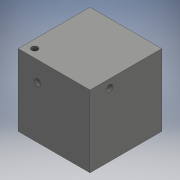
# Autodesk Inventor part: Bundhjørne1
Saved by Autodesk Inventor 2018 (Build 220112000, 112)
## iProperties
Created: 2018-01-29
Part Number: Bundhjørne1
Material: PC/ABS Plastic
Document SubType Name: Modeling
Designer: MikkelS
Density: 0.357273 g/cm^3
Appearance: Smooth - White
Author: MikkelS
Autodesk Inventor part; units mm, degrees
ref_plane "YZ Plane" through (0, 0, 0) normal (1, 0, 0) x (0, 1, 0)
ref_plane "XZ Plane" through (0, 0, 0) normal (0, 1, 0) x (-1, 0, 0)
ref_plane "XY Plane" through (0, 0, 0) normal (0, 0, 1) x (1, 0, 0)
sketch "Sketch1" plane through (0, 0, 0) normal (0, 0, 1) x (1, 0, 0)
  line L0 (0, 0) -> (0, 70)
  line L1 (0, 70) -> (70, 70)
  line L2 (70, 70) -> (70, 0)
  line L3 (70, 0) -> (0, 0)
  dimension "d0" = 70
  dimension "d1" = 70
  constraints: 8 end point, 2 perpendicular, 2 vertical
  measures "d0" distance of L0.start L0.end
  measures "d1" distance of L0.end L1.end
extrude "Extrusion1" add sketch "Sketch1" along normal blind 70
sketch "Sketch2" plane through (0, 0, 70) normal (0, 0, 1) x (1, 0, 0)
  circle A0 centre (8, 8) radius 3
  dimension "d6" = 6
  constraints: 1 centre point
  measures "d6" diameter of A0
hole "Hole1" at (8, 8, 70) direction (0, 0, -1) diameter 6 end through all
sketch "Sketch3" plane through (0, 0, 0) normal (-1, 0, 0) x (0, 0, 1)
  line L0 (69.699, 0) -> (70, 18.9976)
  line L1 (70, 70) -> (70, 0) projected
  line L2 (70, 18.9976) -> (62.001, 19.1244)
  circle A0 centre (62.001, 19.1244) radius 3
  point P0 (0, 0)
  dimension "d14" = 19
  dimension "d15" = 8
  dimension "d16" = 6
  constraints: 4 end point, 1 centre point, 1 coincident, 1 perpendicular, 1 point on line
  measures "d14" distance of L0.start L0.end
  measures "d15" distance of L0.end L2.end
  measures "d16" diameter of A0
hole "Hole2" at (0, 19.1244, 62.001) direction (1, 0, 0) diameter 6 end through all
sketch "Sketch4" plane through (0, 70, 0) normal (0, 1, 0) x (1, 0, 0)
  line L0 (0, -70.1804) -> (0, -51.1804)
  line L1 (0, 0) -> (0, -70) projected
  line L2 (0, -51.1804) -> (19, -51.1804)
  circle A0 centre (19, -51.1804) radius 3
  dimension "d24" = 19
  dimension "d25" = 19
  dimension "d26" = 6
  constraints: 4 end point, 1 centre point, 1 coincident, 1 perpendicular, 1 point on line
  measures "d24" distance of L0.start L0.end
  measures "d25" distance of L0.end L2.end
  measures "d26" diameter of A0
hole "Hole3" at (19, 70, 51.1804) direction (0, -1, 0) diameter 6 end through all
body "Solid1"
